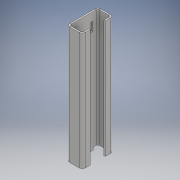
# Autodesk Inventor part: Cprofiel
Saved by Autodesk Inventor 2017 (Build 210142000, 142)
## iProperties
Created: 2017-01-07
Part Number: Cprofiel
Material: Generic
Document SubType Name: Sheet Metal
Designer: bramp
Density: 1 g/cm^3
Sheet Metal Rule: Default_mm
Appearance: Default
Author: bramp
Autodesk Inventor part; units mm, degrees
ref_plane "YZ Plane" through (0, 0, 0) normal (1, 0, 0) x (0, 1, 0)
ref_plane "XZ Plane" through (0, 0, 0) normal (0, 1, 0) x (-1, 0, 0)
ref_plane "XY Plane" through (0, 0, 0) normal (0, 0, 1) x (1, 0, 0)
sketch "Sketch1" plane through (0, 0, 0) normal (0, 0, 1) x (1, 0, 0)
  line L0 (0, 0) -> (-29, 0)
  line L1 (-29, 0) -> (-29, -64)
  line L2 (-29, -64) -> (0, -64)
  line L3 (0, -64) -> (0, -49)
  line L4 (0, 0) -> (0, -15)
  dimension "d0" = 64
  dimension "d1" = 29
  dimension "d2" = 29
  dimension "d13" = 15
  dimension "d14" = 15
  measures "d0" distance between parallel lines of L0 L2
  measures "d1" distance of L0.start L0.end
  measures "d2" distance of L1.end L2.end
  measures "d13" distance of L2.end L3.end
  measures "d14" distance of L0.start L4.end
contour flange "Contour Flange1" sketch "Sketch1" thickness 3 bend radius 3.9 width 265 along (0, 0, 1) mid plane no both sides no wall seen from (0, -7.5, 0) lies toward (1, 0, 0) curves L4 L0 L1 L2 L3
bend "Bend1"
corner "Corner1"
sketch "Sketch2" plane through (-29, -60.1, 0) normal (1, 0, 0) x (0, 0, -1)
  line L0 (0, 0) -> (-265, 0)
  line L1 (0, 56.2) -> (0, 0)
  line L2 (0, 56.2) -> (-265, 56.2)
  line L3 (-265, 0) -> (-265, 56.2)
  line L4 (-265, -6.9) -> (0, -6.9)
  line L5 (-265, -6.9) -> (0, -6.9)
  line L6 (-265, 56.2) -> (0, 56.2)
  line L7 (0, 60.1) -> (-265, 60.1)
  line L8 (-265, 63.1) -> (0, 63.1)
  line L9 (-265, 63.1) -> (0, 63.1)
  line L10 (0, 56.2) -> (0, 0)
  line L11 (0, 6.1) -> (6, 6.1)
  line L12 (6, 6.1) -> (6, 50.1)
  line L13 (6, 50.1) -> (0, 50.1)
  line L14 (0, 50.1) -> (0, 6.1)
  line L15 (0, -3.9) -> (-265, -3.9)
  dimension "d15" = 6
  dimension "d16" = 10
  dimension "d17" = 10
  measures "d15" distance of L13.end L12.end
  measures "d16" distance between parallel lines of L11 L15
  measures "d17" distance between parallel lines of L13 L7
sheet face with bend "Face1" sketch "Sketch2" thickness 3 toward (-1, 0, 0) bend radius 3.9 relief straight relief width 3 relief depth 1.5 contours L1 L13 L12 L11
bend "Bend2"
sketch "Sketch3" plane through (-32, -60.1, 265) normal (-1, 0, 0) x (0, 0, 1)
  line L0 (-18.5, 48.6) -> (-39, 48.6)
  line L1 (-39, 48.6) -> (-39, 44.6)
  line L2 (-39, 44.6) -> (-18.5, 44.6)
  line L3 (-18.5, 44.6) -> (-18.5, 48.6)
  line L4 (-18.5, 11.6) -> (-39, 11.6)
  line L5 (-39, 11.6) -> (-39, 7.6)
  line L6 (-39, 7.6) -> (-18.5, 7.6)
  line L7 (-18.5, 7.6) -> (-18.5, 11.6)
  line L8 (0, 0) -> (-265, 0) projected
  line L9 (0, 56.2) -> (0, 0) projected
  line L10 (0, 56.2) -> (-265, 56.2) projected
  line L11 (-265, 56.2) -> (-265, 50.1) projected
  line L12 (-271, 50.1) -> (-265, 50.1) projected
  line L13 (-271, 6.1) -> (-271, 50.1) projected
  line L14 (-265, 6.1) -> (-271, 6.1) projected
  line L15 (-265, 6.1) -> (-265, 0) projected
  line L16 (0, 0) -> (0, 56.2) projected
  line L17 (0, 28.1) -> (-271, 28.1) construction
  circle A0 centre (-35, 28.1) radius 4.5
  point P0 (-265, 60.1)
  dimension "d33" = 20.5
  dimension "d34" = 20.5
  dimension "d35" = 4
  dimension "d36" = 4
  dimension "d37" = 33
  dimension "d38" = 16.5
  dimension "d40" = 9
  dimension "d41" = 4
  constraints: 18 end point, 5 parallel, 3 point on line, 2 horizontal, 2 midpoint, 2 perpendicular, 1 centre point
  measures "d33" distance between parallel lines of L1 L3
  measures "d34" distance between parallel lines of L7 L5
  measures "d35" distance between parallel lines of L2 L0
  measures "d36" distance between parallel lines of L6 L4
  measures "d37" distance between parallel lines of L4 L2
  measures "d38" distance between parallel lines of L4 L17
  measures "d40" diameter of A0
  measures "d41" distance from line of L1 A0.centre
extrude "Cut1" cut sketch "Sketch3" against normal blind 3 contours L3 L2 L1 L0 | L7 L6 L5 L4 | A0
equation "\"d2\" = d1"
equation "\"d14\" = d13"
equation "\"d36\" = d35"
equation "\"d38\" = 0.5 * d37"
equation "\"d42\" = Thickness"
equation "\"d3\" = BendReliefWidth"
equation "\"d4\" = BendReliefDepth"
equation "\"d5\" = MinimumRemnant"
equation "\"d6\" = BendRadius"
equation "\"d8\" = BendRadius"
equation "\"d10\" = CornerReliefSize"
equation "\"d11\" = GapSize"
equation "\"d12\" = JacobiRadiusSize"
equation "\"d18\" = BendRadius"
equation "\"d19\" = BendReliefWidth"
equation "\"d21\" = MinimumRemnant"
equation "\"d20\" = BendReliefDepth"
equation "\"d22\" = BendRadius"
equation "\"BendReliefWidth\" = Thickness"
equation "\"BendReliefDepth\" = 0.5 * Thickness"
equation "\"CornerReliefSize\" = 4 * Thickness"
equation "\"MinimumRemnant\" = 2 * Thickness"
equation "\"TransitionRadius\" = BendRadius"
equation "\"JacobiRadiusSize\" = BendRadius"
equation "\"GapSize\" = Thickness"
equation "\"Thickness\" = 3"
equation "\"BendRadius\" = 3.9"
body "Solid1"
